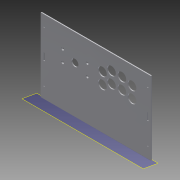
# Autodesk Inventor part: Panel_top_2
Saved by Autodesk Inventor 2013 (Build 170138000, 138)
## iProperties
Created: 2013-01-09
Part Number: Panel_top_2
Material: Aluminum
Document SubType Name: Modeling
Designer: mstine
Density: 1 g/cm^3
Author: mstine
Autodesk Inventor part; units mm, degrees
ref_plane "YZ Plane" through (0, 0, 0) normal (1, 0, 0) x (0, 1, 0)
ref_plane "XZ Plane" through (0, 0, 0) normal (0, 1, 0) x (-1, 0, 0)
ref_plane "XY Plane" through (0, 0, 0) normal (0, 0, 1) x (1, 0, 0)
sketch "Panel" plane through (0, 0, 0) normal (0, 0, 1) x (1, 0, 0)
  line L0 (-190.5, 127) -> (190.5, 127)
  line L1 (190.5, 127) -> (190.5, -127)
  line L2 (190.5, -127) -> (-190.5, -127)
  line L3 (-190.5, -127) -> (-190.5, 127)
  point P0 (0, 0)
  point P1 (-190.5, 0)
  point P2 (0, 127)
  dimension "d0" = 254
  dimension "d3" = 381
  constraints: 8 end point, 2 midpoint, 2 parallel, 1 horizontal, 1 horizontal alignment, 1 perpendicular, 1 vertical alignment
  measures "d0" distance of L2.end L0.start
  measures "d3" distance of L0.start L0.end
sketch "JoystickMount" plane through (0, 0, 0) normal (0, 0, 1) x (1, 0, 0)
  line L0 (-114.625, 55.25) -> (-114.625, 14.75) construction
  line L1 (-114.625, 14.75) -> (-29.625, 14.75) construction
  point P0 (0, 0)
  point P1 (-72.125, 35)
  point P2 (-29.625, 55.25)
  point P3 (-114.625, 35)
  point P4 (-72.125, 14.75)
  dimension "d4" = 40.5
  dimension "d6" = 85
  dimension "d19" = 35
  dimension "d45" = 72.125
  constraints: 4 end point, 3 horizontal alignment, 3 vertical alignment, 2 midpoint, 1 perpendicular, 1 vertical
  measures "d4" distance of L0.start L0.end
  measures "d6" distance of L0.end L1.end
  measures "d19" vertical distance of point (0, 0) point (-72.125, 35)
  measures "d45" horizontal distance of point (0, 0) point (-72.125, 35)
sketch "ButtonMounts" plane through (0, 0, 0) normal (0, 0, 1) x (1, 0, 0)
  line L0 (54.125, 74) -> (54.125, 35) construction
  line L1 (54.125, 35) -> (90.125, 35) construction
  point P0 (0, 0)
  point P1 (22.875, 56)
  point P2 (22.875, 17)
  point P3 (90.125, 74)
  point P4 (125.125, 65)
  point P5 (125.125, 26)
  point P6 (-72.125, 35)
  point P7 (72.125, 54.5)
  point P8 (54.125, 54.5)
  point P9 (72.125, 35)
  dimension "d7" = 39
  dimension "d9" = 39
  dimension "d10" = 39
  dimension "d11" = 39
  dimension "d12" = 31.25
  dimension "d13" = 36
  dimension "d14" = 35
  dimension "d15" = 18
  dimension "d16" = 9
  dimension "d55" = 144.25
  dimension "d56" = 72.125
  constraints: 5 vertical alignment, 4 end point, 3 horizontal alignment, 2 midpoint
  measures "d7" distance of point (22.875, 17) point (22.875, 56)
  measures "d9" distance of L0.start L0.end
  measures "d10" distance of L1.end point (90.125, 74)
  measures "d11" distance of point (125.125, 26) point (125.125, 65)
  measures "d12" horizontal distance of L0.end point (22.875, 17)
  measures "d13" distance of L0.end L1.end
  measures "d14" horizontal distance of L1.end point (125.125, 26)
  measures "d15" vertical distance of point (22.875, 17) L0.end
  measures "d16" vertical distance of point (125.125, 26) L1.end
  measures "d55" horizontal distance of point (72.125, 54.5) point (-72.125, 35)
  measures "d56" horizontal distance of point (72.125, 54.5) point (0, 0)
extrude "PanelExtrusion" add sketch "Panel" against normal blind 3.175
hole "JoystickScrews" at (-29.625, 14.75, 0) at (-29.625, 55.25, 0) at (-114.625, 55.25, 0) at (-114.625, 14.75, 0) direction (0, 0, -1) diameter 4.5 end through all countersink diameter 9.4 countersink angle 90 clearance for "Flat Head Machine Screw" size "M4" standard "Ansi Metric M Profile"
hole "JoystickShaft" at (-72.125, 35, 0) direction (0, 0, -1) diameter 24 end through all
hole "ButtonHoles" at (125.125, 26, 0) at (90.125, 35, 0) at (90.125, 74, 0) at (125.125, 65, 0) at (54.125, 74, 0) at (54.125, 35, 0) at (22.875, 56, 0) at (22.875, 17, 0) direction (0, 0, -1) diameter 30 end through all
fillet "Corners" radius 1 4 edges at (190.5, 127, -1.5875) (190.5, -127, -1.5875) (-190.5, 127, -1.5875) (-190.5, -127, -1.5875)
ref_plane "10DegOffsetAlignment" through (190.5, -127, -3.175) normal (0, -0.9848078, 0.1736482) x (-1, 0, 0)
sketch "ScrewHoleCenters" plane through (0, 0, 0) normal (0, 0, 1) x (1, 0, 0)
  line L0 (-190.5, -126) -> (-190.5, 126) projected
  line L1 (-177.8, 89.411) -> (-180.975, 89.411) projected
  line L2 (-180.975, 85.6137) -> (-177.8, 85.6137) projected
  line L3 (-177.8, -85.9663) -> (-180.975, -85.9663) projected
  line L4 (-180.975, -89.7636) -> (-177.8, -89.7636) projected
  line L5 (177.8, -89.7636) -> (180.975, -89.7636) projected
  line L6 (180.975, -85.9663) -> (177.8, -85.9663) projected
  line L7 (177.8, 85.6137) -> (180.975, 85.6137) projected
  line L8 (180.975, 89.411) -> (177.8, 89.411) projected
  line L9 (-180.975, 89.411) -> (-180.975, 85.6137) construction
  line L10 (-177.8, 85.6137) -> (-177.8, 89.411) construction
  line L11 (-180.975, -85.9663) -> (-180.975, -89.7636) construction
  line L12 (-177.8, -89.7636) -> (-177.8, -85.9663) construction
  line L13 (177.8, -89.7636) -> (177.8, -85.9663) construction
  line L14 (180.975, -85.9663) -> (180.975, -89.7636) construction
  line L15 (177.8, 85.6137) -> (177.8, 89.411) construction
  line L16 (180.975, 89.411) -> (180.975, 85.6137) construction
  point P0 (0, 0)
  point P1 (-179.3875, 87.5123)
  point P2 (-177.8, 87.5123)
  point P3 (-179.3875, 85.6137)
  point P4 (-179.3875, -87.865)
  point P5 (179.3875, -87.865)
  point P6 (179.3875, 87.5123)
  point P7 (-179.3875, -89.7636)
  point P8 (-180.975, -87.865)
  point P9 (177.8, -87.865)
  point P10 (179.3875, -89.7636)
  point P11 (179.3875, 85.6137)
  point P12 (177.8, 87.5123)
  constraints: 16 end point, 8 midpoint, 8 parallel, 4 horizontal alignment, 4 vertical alignment
hole "PanelBoltHoles" at (-179.3875, 87.5123, 0) at (-179.3875, -87.865, 0) at (179.3875, -87.865, 0) at (179.3875, 87.5123, 0) direction (0, 0, -1) diameter 3.7973 end through all
sketch "TabSlotSketch" plane through (0, 0, 0) normal (0, 0, 1) x (1, 0, 0)
  circle A0 centre (179.3875, -87.865) radius 1.8986 projected
  circle A1 centre (-179.3875, 87.5123) radius 1.8986 projected
  circle A2 centre (-179.3875, -87.865) radius 1.8986 projected
  circle A3 centre (179.3875, 87.5123) radius 1.8986 projected
  line L0 (190.5, 126) -> (190.5, -126) projected
  line L1 (-190.5, -126) -> (-190.5, 126) projected
  line L2 (-179.3875, 87.5123) -> (-179.3875, -87.865) construction
  line L3 (179.3875, 87.5123) -> (179.3875, -87.865) construction
  line L4 (-181.2925, 12.5237) -> (-177.4825, 12.5237)
  line L5 (-177.4825, 12.5237) -> (-177.4825, -12.8763)
  line L6 (-177.4825, -12.8763) -> (-181.2925, -12.8763)
  line L7 (-181.2925, -12.8763) -> (-181.2925, 12.5237)
  line L8 (181.2925, -12.8763) -> (177.4825, -12.8763)
  line L9 (177.4825, -12.8763) -> (177.4825, 12.5237)
  line L10 (177.4825, 12.5237) -> (181.2925, 12.5237)
  line L11 (181.2925, 12.5237) -> (181.2925, -12.8763)
  point P0 (0, 0)
  point P1 (-179.3875, -0.1763)
  point P2 (-181.2925, -0.1763)
  point P3 (-179.3875, -12.8763)
  point P4 (179.3875, -0.1763)
  point P5 (181.2925, -0.1763)
  point P6 (179.3875, 12.5237)
  point P7 (-179.3875, -0.1763)
  point P8 (179.3875, -0.1763)
  dimension "d66" = 25.4
  dimension "d68" = 3.81
  dimension "d69" = 25.4
  dimension "d70" = 3.81
  constraints: 20 end point, 6 midpoint, 6 parallel, 2 coincident, 2 horizontal, 2 horizontal alignment, 2 perpendicular, 2 vertical alignment
  measures "d66" distance of L4.end L5.end
  measures "d68" distance of L4.start L4.end
  measures "d69" distance of L10.end L8.start
  measures "d70" distance of L9.end L10.end
extrude "TabSlotExtrusion" cut sketch "TabSlotSketch" against normal blind 3.175 contours L4 L5 L6 L7 | L8 L9 L10 L11
fillet "Fillet2" radius 0.5 8 edges at (-177.4825, 12.5237, -1.5875) (-181.2925, 12.5237, -1.5875) (-177.4825, -12.8763, -1.5875) (-181.2925, -12.8763, -1.5875) (181.2925, 12.5237, -1.5875) (177.4825, 12.5237, -1.5875) (177.4825, -12.8763, -1.5875) (181.2925, -12.8763, -1.5875)
equation "\"d45\" = 0.5 * d55"
equation "\"d59\" = ScrewHoleD"
equation "\"d66\" = SlotLength"
equation "\"d68\" = SlotWidth"
equation "\"d69\" = SlotLength"
equation "\"d70\" = SlotWidth"
equation "\"d73\" = SlotFilletRad"
equation "\"SlotLength\" = 25.4"
equation "\"ScrewHoleD\" = 3.7973"
equation "\"SlotWidth\" = 3.81"
equation "\"SlotFilletRad\" = 0.5"
